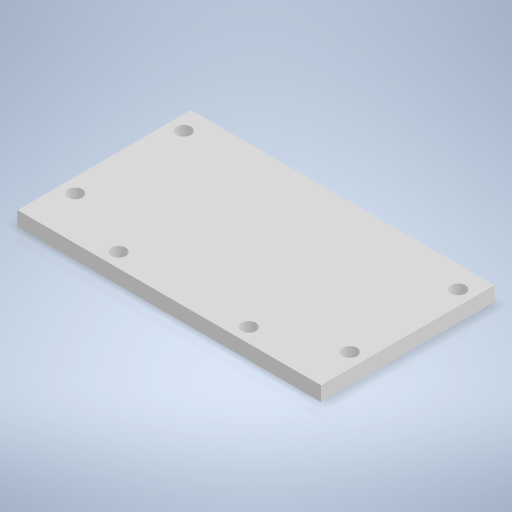
# Autodesk Inventor part: 1012
Saved by Autodesk Inventor 2024 (Build 280153000, 153)
## iProperties
Created: 2024-07-12
Part Number: 1012
Material: Generisch
Document SubType Name: Modeling
Designer: ffogue
Density: 1 g/cm^3
Appearance: Vorgabe
Author: ffogue
Autodesk Inventor part; units mm, degrees
ref_plane "YZ Plane" through (0, 0, 0) normal (1, 0, 0) x (0, 1, 0)
ref_plane "XZ Plane" through (0, 0, 0) normal (0, 1, 0) x (-1, 0, 0)
ref_plane "XY Plane" through (0, 0, 0) normal (0, 0, 1) x (1, 0, 0)
sketch "Skizze1" plane through (0, 0, 0) normal (0, 0, 1) x (1, 0, 0)
  line L0 (0, 0) -> (84, 0)
  line L1 (84, 0) -> (84, 48)
  line L2 (84, 48) -> (0, 48)
  line L3 (0, 48) -> (0, 0)
  dimension "d0" = 48
  dimension "d1" = 84
  constraints: 8 end point, 2 parallel, 1 horizontal, 1 perpendicular
  measures "d0" distance between parallel lines of L0 L2
  measures "d1" distance between parallel lines of L1 L3
extrude "Extrusion1" add sketch "Skizze1" along normal blind 4
sketch "Skizze2" plane through (0, 0, 4) normal (0, 0, 1) x (1, 0, 0)
  line L0 (0, 48) -> (0, 0) projected
  line L1 (0, 0) -> (84, 0) projected
  line L2 (84, 0) -> (84, 48) projected
  point P0 (4, 12)
  point P1 (4, 42)
  point P2 (80, 42)
  point P3 (80, 12)
  dimension "d4" = 4
  dimension "d5" = 30
  dimension "d6" = 12
  dimension "d7" = 4
  constraints: 2 horizontal alignment, 2 vertical alignment
  measures "d4" distance from line of L0 point (4, 12)
  measures "d5" distance of point (4, 12) point (4, 42)
  measures "d6" distance from line of L1 point (4, 12)
  measures "d7" distance from line of L2 point (80, 12)
hole "Bohrung1" at (4, 12, 4) at (4, 42, 4) at (80, 42, 4) at (80, 12, 4) direction (0, 0, -1) diameter 4 depth 4
sketch "Skizze3" plane through (0, 0, 4) normal (0, 0, 1) x (1, 0, 0)
  line L0 (0, 0) -> (84, 0) projected
  line L1 (0, 48) -> (0, 0) projected
  point P0 (24, 4)
  point P1 (60, 4)
  dimension "d15" = 4
  dimension "d16" = 24
  dimension "d17" = 36
  constraints: 1 horizontal alignment
  measures "d15" distance from line of L0 point (24, 4)
  measures "d16" distance from line of L1 point (24, 4)
  measures "d17" distance of point (60, 4) point (24, 4)
hole "Bohrung2" at (24, 4, 4) at (60, 4, 4) direction (0, 0, -1) diameter 4 depth 4
equation "\"d7\" = d4"
